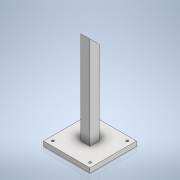
# Autodesk Inventor part: Viewing Mirror Holder
Saved by Autodesk Inventor 2022 (Build 260153000, 153)
## iProperties
Created: 2023-09-18
Part Number: Viewing Mirror Holder
Material: Generic
Document SubType Name: Modeling
Designer: fouad
Density: 1 g/cm^3
Appearance: Default
Author: fouad
Autodesk Inventor part; units mm, degrees
ref_plane "YZ Plane" through (0, 0, 0) normal (1, 0, 0) x (0, 1, 0)
ref_plane "XZ Plane" through (0, 0, 0) normal (0, 1, 0) x (-1, 0, 0)
ref_plane "XY Plane" through (0, 0, 0) normal (0, 0, 1) x (1, 0, 0)
sketch "Sketch2" plane through (0, 0, 0) normal (0, 1, 0) x (-1, 0, 0)
  line L0 (2.5667, 3.1167) -> (0.5667, 3.1167)
  line L1 (0.5667, 3.1167) -> (0.5667, 1.1167)
  line L2 (0.5667, 1.1167) -> (2.5667, 1.1167)
  line L3 (2.5667, 1.1167) -> (2.5667, 3.1167)
  point P0 (0, 0)
  dimension "d5" = 2
  dimension "d6" = 2
  constraints: 8 end point, 2 parallel, 1 horizontal, 1 perpendicular
  measures "d5" distance of L2.end L1.end
  measures "d6" distance of L1.end L0.end
extrude "Extrusion1" add sketch "Sketch2" along normal blind 20
sketch "Sketch3" plane through (-0.5667, 0, 3.1167) normal (1, 0, 0) x (0, 0, -1)
  line L0 (0, 20) -> (2, 20) projected
  line L1 (0, 20) -> (2, 18)
  line L2 (2, 0) -> (2, 20) projected
  line L3 (0, 20) -> (2.8284, 20) construction
  point P0 (3.1167, 0)
  dimension "d9" = 45
  constraints: 4 end point, 1 equal length, 1 horizontal, 1 point on line
  measures "d9" angle of L1 L3
extrude "Extrusion2" cut sketch "Sketch3" against normal through all
sketch "Sketch4" plane through (0, 0, 0) normal (0, -1, 0) x (1, 0, 0)
  line L0 (3.4333, 7.1167) -> (-6.5667, 7.1167)
  line L1 (-6.5667, 7.1167) -> (-6.5667, -2.8833)
  line L2 (-6.5667, -2.8833) -> (3.4333, -2.8833)
  line L3 (3.4333, -2.8833) -> (3.4333, 7.1167)
  line L4 (-2.5667, 1.1167) -> (-2.5667, 3.1167) projected
  line L5 (-0.5667, 1.1167) -> (-2.5667, 1.1167) projected
  point P0 (0, 0)
  dimension "d12" = 10
  dimension "d13" = 10
  dimension "d14" = 4
  dimension "d15" = 4
  constraints: 8 end point, 2 parallel, 1 horizontal, 1 perpendicular
  measures "d12" distance of L2.end L1.end
  measures "d13" distance of L1.end L0.end
  measures "d14" distance between parallel lines of L4 L1
  measures "d15" distance between parallel lines of L5 L2
extrude "Extrusion3" add sketch "Sketch4" along normal blind 1
sketch "Sketch5" plane through (0, 0, 0) normal (0, 1, 0) x (1, 0, 0)
  circle A0 centre (-5.5667, 1.8833) radius 0.25
  line L0 (-6.5667, -7.1167) -> (-6.5667, 2.8833) projected
  line L1 (3.4333, 2.8833) -> (3.4333, -7.1167) projected
  line L2 (-6.5667, 2.8833) -> (3.4333, 2.8833) projected
  circle A1 centre (-5.5667, -6.1167) radius 0.25
  circle A2 centre (2.4333, 1.8833) radius 0.25
  circle A3 centre (2.4333, -6.1167) radius 0.25
  point P0 (0, 0)
  dimension "d18" = 0.5
  dimension "d20" = 9
  dimension "d22" = 1
  dimension "d25" = 8
  dimension "d28" = 8
  constraints: 4 centre point, 1 horizontal, 1 vertical, 6 other
  measures "d18" diameter of A0
  measures "d20" distance from line of A0.centre L1
  measures "d22" distance from line of A0.centre L2
  measures "d25" distance of A0.centre A1.centre
  measures "d28" distance of A0.centre A2.centre
extrude "Extrusion4" cut sketch "Sketch5" against normal through all
body "Solid1"
